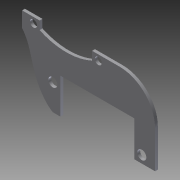
# Autodesk Inventor part: Dewalt Drill Drive Servo Shift Mount Plate
Saved by Autodesk Inventor 2012 (Build 160160000, 160)
## iProperties
Created: 2012-07-04
Part Number: Dewalt Drill Drive Servo Shift Mount Plate
Material: Default
Document SubType Name: Modeling
Designer: Bruce
Density: 1 g/cm^3
Author: Bruce
Autodesk Inventor part; units mm, degrees
ref_plane "YZ Plane" through (0, 0, 0) normal (1, 0, 0) x (0, 1, 0)
ref_plane "XZ Plane" through (0, 0, 0) normal (0, 1, 0) x (-1, 0, 0)
ref_plane "XY Plane" through (0, 0, 0) normal (0, 0, 1) x (1, 0, 0)
sketch "Sketch1" plane through (0, 0, 0) normal (0, 0, 1) x (1, 0, 0)
  line L0 (-71.374, 39.116) -> (0, 39.116)
  line L1 (0, 39.116) -> (0, 0)
  line L2 (0, 0) -> (-54.864, 0)
  line L3 (-71.374, 0) -> (-71.374, 39.116)
  line L4 (-50.8, 19.05) -> (-11.176, 19.05)
  line L5 (-11.176, 19.05) -> (-11.176, 0)
  line L6 (-11.176, 0) -> (-50.8, 0)
  line L7 (-50.8, 0) -> (-50.8, 19.05)
  line L8 (-61.976, 39.116) -> (-33.782, 39.116)
  line L9 (-33.782, 39.116) -> (-33.782, 34.5451)
  line L10 (-61.976, 34.5421) -> (-61.976, 39.116)
  arc A0 (-61.976, 34.6628) -> (-33.782, 34.5451) centre (-47.752, 65.024) ccw
  circle A1 centre (-7.112, 4.064) radius 2.4384
  circle A2 centre (-54.864, 13.97) radius 2.4384
  circle A3 centre (-65.278, 36.068) radius 1.905
  circle A4 centre (-30.48, 36.068) radius 1.905
  spline S0 degree 4 poles (-71.374, 30.861) (-64.6272, 22.5308) (-68.0392, 14.6486) (-60.5114, 2.9461) (-54.864, 0) knots 0 0 0 0 0 1 1 1 1 1
  line L11 (-54.864, 0) -> (-71.374, 0)
  point P0 (-64.4411, 13.1063)
  point P1 (-59.9147, 4.6412)
  dimension "d0" = 71.374
  dimension "d1" = 39.116
  dimension "d2" = 11.176
  dimension "d3" = 50.8
  dimension "d4" = 19.05
  dimension "d5" = 65.024
  dimension "d6" = 47.752
  dimension "d7" = 33.782
  dimension "d8" = 61.976
  dimension "d9" = 33.528
  dimension "d10" = 4.8768
  dimension "d11" = 4.8768
  dimension "d12" = 7.112
  dimension "d13" = 4.064
  dimension "d14" = 54.864
  dimension "d15" = 13.97
  dimension "d16" = 3.81
  dimension "d17" = 3.81
  dimension "d18" = 36.068
  dimension "d19" = 30.48
  dimension "d20" = 65.278
  dimension "d21" = 8.255
  constraints: 24 end point, 6 parallel, 5 centre point, 4 point on line, 3 horizontal, 3 perpendicular, 2 coincident, 2 point on circle, 1 horizontal alignment, 1 vertical alignment, 6 other
  measures "d0" distance of L0.start L0.end
  measures "d1" distance of L0.end L1.end
  measures "d2" distance between parallel lines of L1 L5
  measures "d3" distance between parallel lines of L1 L7
  measures "d4" distance between parallel lines of L2 L4
  measures "d5" distance from line of L2 point (-47.752, 65.024)
  measures "d6" distance from line of L1 point (-47.752, 65.024)
  measures "d7" distance between parallel lines of L1 L9
  measures "d8" distance between parallel lines of L1 L10
  measures "d9" radius of A0
  measures "d10" diameter of A1
  measures "d11" diameter of A2
  measures "d12" distance from line of L1 A1.centre
  measures "d13" distance from line of L2 A1.centre
  measures "d14" distance from line of L1 A2.centre
  measures "d15" distance from line of L6 A2.centre
  measures "d16" diameter of A4
  measures "d17" diameter of A3
  measures "d18" distance from line of L2 A4.centre
  measures "d19" distance from line of A4.centre L1
  measures "d20" distance from line of L1 A3.centre
  measures "d21" distance from line of point (-71.374, 30.861) L0
extrude "Extrusion1" add sketch "Sketch1" against normal blind 1.524 contours L0 L10 A0 L9 L1 L2 L5 L4 L7 S0 L3
fillet "Fillet1" radius 19.05 1 edges at (0, 39.116, -0.762)
equation "\"d11\" = d10"
equation "\"d17\" = d16"
body "Solid1"
